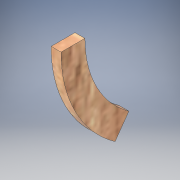
# Autodesk Inventor part: Speaker Clamp Back
Saved by Autodesk Inventor 2018 (Build 220112000, 112)
## iProperties
Created: 2017-12-07
Part Number: Speaker Clamp Back
Material: Wood (Birch)
Document SubType Name: Modeling
Designer: Andrew
Density: 0.55 g/cm^3
Appearance: Birch - Natural Polished
Author: Andrew
Autodesk Inventor part; units mm, degrees
ref_plane "YZ Plane" through (0, 0, 0) normal (1, 0, 0) x (0, 1, 0)
ref_plane "XZ Plane" through (0, 0, 0) normal (0, 1, 0) x (-1, 0, 0)
ref_plane "XY Plane" through (0, 0, 0) normal (0, 0, 1) x (1, 0, 0)
derived "Speaker Clamp.ipt"
sketch "Sketch1" plane through (3.302, -56.7835, 90.4875) normal (1, 0, 0) x (0, 0, -1)
  circle A0 centre (41.275, 18.5565) radius 28.575 construction
  line L0 (24.4552, 53.4815) -> (-3.302, 53.4815)
  line L1 (0, 25.75) -> (0, 0)
  line L2 (16.3225, 23.3034) -> (36.5281, 43.509) construction
  line L3 (14.0774, 25.5485) -> (34.283, 45.754)
  line L4 (38.7731, 41.2639) -> (18.5676, 21.0583)
  arc A1 (14.0774, 25.5485) -> (18.5676, 21.0583) centre (16.3225, 23.3034) ccw
  arc A2 (38.7731, 41.2639) -> (34.283, 45.754) centre (36.5281, 43.509) ccw
  line L5 (17.4962, 9.6274) -> (50.2041, 42.3353) construction
  line L6 (15.2511, 11.8725) -> (47.959, 44.5804)
  line L7 (52.4492, 40.0902) -> (19.7413, 7.3823)
  arc A3 (15.2511, 11.8725) -> (19.7413, 7.3823) centre (17.4962, 9.6274) ccw
  arc A4 (52.4492, 40.0902) -> (47.959, 44.5804) centre (50.2041, 42.3353) ccw
  line L8 (23.3145, 0.596) -> (59.2355, 36.517) construction
  line L9 (21.0694, 2.841) -> (56.9904, 38.7621)
  line L10 (61.4806, 34.2719) -> (25.5596, -1.6491)
  arc A5 (21.0694, 2.841) -> (25.5596, -1.6491) centre (23.3145, 0.596) ccw
  arc A6 (61.4806, 34.2719) -> (56.9904, 38.7621) centre (59.2355, 36.517) ccw
  line L11 (32.3459, -5.2223) -> (65.0538, 27.4856) construction
  line L12 (30.1008, -2.9772) -> (62.8087, 29.7307)
  line L13 (67.2989, 25.2405) -> (34.591, -7.4674)
  arc A7 (30.1008, -2.9772) -> (34.591, -7.4674) centre (32.3459, -5.2223) ccw
  arc A8 (67.2989, 25.2405) -> (62.8087, 29.7307) centre (65.0538, 27.4856) ccw
  line L14 (46.0219, -6.396) -> (66.2275, 13.8096) construction
  line L15 (48.267, -8.6411) -> (68.4726, 11.5645)
  line L16 (63.9824, 16.0546) -> (43.7769, -4.1509)
  arc A9 (43.7769, -4.1509) -> (48.267, -8.6411) centre (46.0219, -6.396) ccw
  arc A10 (68.4726, 11.5645) -> (63.9824, 16.0546) centre (66.2275, 13.8096) ccw
  circle A11 centre (41.275, 18.5565) radius 34.925 construction
  circle A12 centre (146.05, 18.5565) radius 3.4925
  circle A13 centre (146.05, 18.5565) radius 19.05 construction
  line L17 (131.1197, 53.4815) -> (103.1875, 53.4815)
  line L18 (180.975, 0) -> (180.975, 25.75)
  line L19 (24.2802, -14.8085) -> (50.0302, -14.8085)
  line L20 (24.2802, -18.3335) -> (24.2802, -14.8085)
  line L21 (50.0302, -18.3335) -> (24.2802, -18.3335)
  line L22 (50.0302, -14.8085) -> (50.0302, -18.3335)
  circle A14 centre (37.1553, 51.9575) radius 1.4605
  point P0 (90.4875, 56.7835)
  point P1 (26.4253, 33.4062)
  point P2 (33.8501, 25.9813)
  point P3 (48.6999, 11.1316)
  point P4 (56.1247, 3.7068)
sketch "Sketch2" plane through (0, 0, 0) normal (1, 0, 0) x (0, 1, 0)
  arc A0 (-38.227, 85.0265) -> (-71.592, 62.2287) centre (-38.227, 49.2125) ccw
  arc A1 (-38.227, 90.1065) -> (-71.592, 72.8577) centre (-38.227, 49.2125) ccw
  line L0 (-38.227, 90.1065) -> (-38.227, 85.0265)
  line L1 (-71.592, 72.8577) -> (-71.592, 62.2287)
  line L2 (-3.302, 66.0323) -> (-3.302, 93.7895)
  line L3 (-71.592, 66.2073) -> (-71.592, 40.4573)
  circle A2 centre (-38.227, 49.2125) radius 34.925 construction
  point P0 (0, 0)
sketch "Sketch3" plane through (0, 0, 0) normal (1, 0, 0) x (0, 1, 0)
  arc A0 (-38.227, 90.1065) -> (-71.592, 72.8577) centre (-38.227, 49.2125) ccw projected
  arc A1 (-38.227, 85.0265) -> (-71.592, 62.2287) centre (-38.227, 49.2125) ccw construction
  arc A2 (-38.227, 82.4865) -> (-65.3749, 68.4518) centre (-38.227, 49.2125) ccw
  line L0 (-38.227, 90.1065) -> (-38.227, 82.4865)
  line L1 (-71.592, 72.8577) -> (-65.3749, 68.4518)
  point P0 (0, 0)
  dimension "d1" = 2.54
  constraints: 4 end point, 2 point on circle, 1 centre point, 1 concentric, 1 point on line, 1 vertical
  measures "d1" radial gap between concentric circles of A1 A2
derived "Wood Rail.ipt"
extrude "Extrusion1" add sketch "Sketch3" along normal blind 3.175
equation "\"d8\" = woodThickness"
equation "\"woodThickness\" = 3.175"
body "Solid1"
